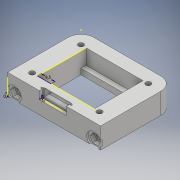
# Autodesk Inventor part: golova 2 prostavka
Saved by Autodesk Inventor 2018.2 (Build 222227000, 227)
## iProperties
Created: 2026-01-20
Part Number: golova 2 prostavka
Material: Типовые
Document SubType Name: Modeling
Designer: Denis
Density: 1 g/cm^3
Appearance: По умолчанию
Author: Denis
## iProperties of the stored document golova 2 prostavka_3DПЕЧАТЬ.ipt
Created: 2026-01-20
Part Number: golova 2 prostavka_3DПЕЧАТЬ
Material: Типовые
Document SubType Name: Modeling
Designer: Denis
Density: 1 g/cm^3
Appearance: По умолчанию
Author: Denis
Autodesk Inventor part; units mm, degrees
ref_plane "YZ Plane" through (0, 0, 0) normal (1, 0, 0) x (0, 1, 0)
ref_plane "XZ Plane" through (0, 0, 0) normal (0, 1, 0) x (-1, 0, 0)
ref_plane "XY Plane" through (0, 0, 0) normal (0, 0, 1) x (1, 0, 0)
sketch "Эскиз1" plane through (0, 0, 0) normal (0, 0, 1) x (1, 0, 0)
  point P0 (0, 0)
sketch "Эскиз2" plane through (0, 0, 0) normal (0, 0, 1) x (1, 0, 0)
  line L0 (0, 0) -> (64.3, 0)
  line L1 (64.3, 0) -> (64.3, -50.7)
  line L2 (64.3, -50.7) -> (0, -50.7)
  line L3 (0, -50.7) -> (0, 0)
  dimension "d0" = 64.3
  dimension "d1" = 50.7
  constraints: 8 end point, 2 parallel, 1 horizontal, 1 perpendicular
  measures "d0" distance of L1.end L2.end
  measures "d1" distance of L0.end L1.end
extrude "Выдавливание1" add sketch "Эскиз2" along normal blind 11.5
sketch "Эскиз3" plane through (0, 0, 11.5) normal (0, 0, 1) x (1, 0, 0)
  line L0 (64.3, 0) -> (0, 0) projected
  line L1 (0, 0) -> (0, -12.4)
  line L2 (0, 0) -> (0, -50.7) projected
  line L3 (0, -12.4) -> (12.4, -12.4)
  line L4 (12.4, -12.4) -> (51.9, -12.4)
  line L5 (51.9, -12.4) -> (51.9, -39.1)
  line L6 (51.9, -39.1) -> (12.4, -39.1)
  line L7 (12.4, -39.1) -> (12.4, -12.4)
  dimension "d4" = 12.4
  dimension "d5" = 12.4
  dimension "d6" = 39.5
  dimension "d7" = 26.7
  constraints: 12 end point, 2 parallel, 2 perpendicular, 1 horizontal, 1 point on line
  measures "d4" distance of L0.end L1.end
  measures "d5" distance of L1.end L3.end
  measures "d6" distance of L5.end L6.end
  measures "d7" distance of L4.end L5.end
extrude "Выдавливание2" cut sketch "Эскиз3" against normal blind 11.5
sketch "Эскиз4" plane through (0, 0, 11.5) normal (0, 0, 1) x (1, 0, 0)
  line L0 (12.4, -39.1) -> (51.9, -39.1) projected
  line L1 (12.4, -39.1) -> (8.8645, -42.6355)
  line L2 (12.4, -39.1) -> (17.4, -39.1) construction
  circle A0 centre (8.8645, -42.6355) radius 1.7
  line L3 (51.9, -12.4) -> (12.4, -12.4) projected
  line L4 (12.4, -12.4) -> (8.8645, -8.8645)
  line L5 (12.4, -12.4) -> (17.4, -12.4) construction
  circle A1 centre (8.8645, -8.8645) radius 1.7
  line L6 (51.9, -39.1) -> (51.9, -12.4) projected
  line L7 (51.9, -12.4) -> (55.4355, -8.8645)
  line L8 (51.9, -12.4) -> (56.9, -12.4) construction
  circle A2 centre (55.4355, -8.8645) radius 1.7
  line L9 (51.9, -39.1) -> (55.4355, -42.6355)
  circle A3 centre (55.4355, -42.6355) radius 1.7
  point P0 (0, 0)
  dimension "d10" = 5
  dimension "d11" = 135
  dimension "d12" = 3.4
  dimension "d13" = 5
  dimension "d14" = 135
  dimension "d15" = 3.4
  dimension "d16" = 5
  dimension "d17" = 45
  dimension "d18" = 3.4
  dimension "d19" = 3.4
  constraints: 14 end point, 4 centre point, 4 coincident, 3 equal length, 3 horizontal
  measures "d10" distance of L0.start L1.end
  measures "d11" angle of L1 L2
  measures "d12" diameter of A0
  measures "d13" distance of L3.end L4.end
  measures "d14" angle of L5 L4
  measures "d15" diameter of A1
  measures "d16" distance of L3.start L7.end
  measures "d17" angle of L8 L7
  measures "d18" diameter of A2
  measures "d19" diameter of A3
extrude "Выдавливание3" cut sketch "Эскиз4" against normal blind 11.5
sketch "Эскиз5" plane through (0, 0, 11.5) normal (0, 0, 1) x (1, 0, 0)
  circle A0 centre (8.8645, -8.8645) radius 1.7 projected
  circle A1 centre (8.8645, -8.8645) radius 1.8
  circle A2 centre (55.4355, -8.8645) radius 1.7 projected
  circle A3 centre (55.4355, -8.8645) radius 1.8
  circle A4 centre (55.4355, -42.6355) radius 1.7 projected
  circle A5 centre (55.4355, -42.6355) radius 1.8
  circle A6 centre (8.8645, -42.6355) radius 1.7 projected
  circle A7 centre (8.8645, -42.6355) radius 1.8
  point P0 (0, 0)
  dimension "d22" = 3.6
  dimension "d23" = 3.6
  dimension "d24" = 3.6
  dimension "d25" = 3.6
  constraints: 4 centre point, 4 coincident
  measures "d22" diameter of A1
  measures "d23" diameter of A3
  measures "d24" diameter of A5
  measures "d25" diameter of A7
extrude "Выдавливание4" cut sketch "Эскиз5" against normal blind 11.5 contours A0 | A3 | A5 | A7
sketch "Эскиз6" plane through (0, 0, 11.5) normal (0, 0, 1) x (1, 0, 0)
  circle A0 centre (8.8645, -8.8645) radius 1.7 projected
  circle A1 centre (8.8645, -8.8645) radius 1.8
  point P0 (0, 0)
  dimension "d28" = 3.6
  constraints: 1 centre point, 1 coincident
  measures "d28" diameter of A1
extrude "Выдавливание5" cut sketch "Эскиз6" against normal blind 11.5 contours A0 | A1
sketch "Эскиз7" plane through (0, 0, 11.5) normal (0, 0, 1) x (1, 0, 0)
  point P0 (0, 0)
sketch "Эскиз8" plane through (0, 0, 11.5) normal (0, 0, 1) x (1, 0, 0)
  line L0 (12.4, -39.1) -> (12.4, -12.4) projected
  line L1 (12.4, -12.4) -> (51.9, -12.4)
  line L2 (51.9, -12.4) -> (51.9, -8.9)
  line L3 (51.9, -8.9) -> (12.4, -8.9)
  line L4 (12.4, -8.9) -> (12.4, -12.4)
  line L5 (51.9, -39.1) -> (12.4, -39.1) projected
  line L6 (12.4, -39.1) -> (51.9, -39.1)
  line L7 (51.9, -39.1) -> (51.9, -42.6)
  line L8 (51.9, -42.6) -> (12.4, -42.6)
  line L9 (12.4, -42.6) -> (12.4, -39.1)
  point P0 (0, 0)
  dimension "d31" = 39.5
  dimension "d32" = 3.5
  dimension "d33" = 39.5
  dimension "d34" = 3.5
  constraints: 16 end point, 4 parallel, 2 horizontal, 2 perpendicular
  measures "d31" distance of L3.end L2.end
  measures "d32" distance of L2.end L1.end
  measures "d33" distance of L7.end L8.end
  measures "d34" distance of L6.end L7.end
extrude "Выдавливание6" cut sketch "Эскиз8" against normal blind 7.5
sketch "Эскиз9" plane through (0, 0, 11.5) normal (0, 0, 1) x (1, 0, 0)
  point P0 (0, 0)
sketch "Эскиз10" plane through (0, 0, 11.5) normal (0, 0, 1) x (1, 0, 0)
  point P0 (0, 0)
fillet "Сопряжение1" radius 9 2 edges at (64.3, 0, 5.75) (0, 0, 5.75)
sketch "Эскиз11" plane through (0, 0, 11.5) normal (0, 0, 1) x (1, 0, 0)
  point P0 (0, 0)
sketch "Эскиз12" plane through (0, -50.7, 0) normal (0, -1, 0) x (1, 0, 0)
  point P0 (0, 0)
sketch "Эскиз13" plane through (0, -50.7, 0) normal (0, -1, 0) x (1, 0, 0)
  line L0 (0, 0) -> (0, 11.5) projected
  line L1 (0, 0) -> (0, 0.6)
  dimension "d38" = 0.6
  constraints: 2 end point, 1 point on line
  measures "d38" distance of L0.start L1.end
sketch "Эскиз14" plane through (0, -50.7, 0) normal (0, -1, 0) x (1, 0, 0)
  line L0 (64.3, 0) -> (0, 0) projected
  line L1 (0, 0) -> (0, 0.8)
  line L2 (0, 0) -> (0, 11.5) projected
  line L3 (0, 0.8) -> (2.8, 0.8)
  line L4 (2.8, 0.8) -> (6.4, 0.8)
  line L5 (6.4, 0.8) -> (8.2, 3.9177)
  line L6 (8.2, 3.9177) -> (6.4, 7.0354)
  line L7 (6.4, 7.0354) -> (2.8, 7.0354)
  line L8 (2.8, 7.0354) -> (1, 3.9177)
  line L9 (1, 3.9177) -> (2.8, 0.8)
  dimension "d39" = 0.8
  dimension "d40" = 2.8
  dimension "d41" = 3.6
  dimension "d42" = 3.6
  dimension "d43" = 120
  dimension "d44" = 3.6
  dimension "d45" = 120
  constraints: 16 end point, 2 parallel, 2 point on line, 1 perpendicular
  measures "d39" distance of L0.end L1.end
  measures "d40" distance of L1.end L3.end
  measures "d41" distance of L3.end L4.end
  measures "d42" distance of L4.end L5.end
  measures "d43" angle of L5 L4
  measures "d44" distance of L5.end L6.end
  measures "d45" angle of L6 L5
extrude "Выдавливание7" cut sketch "Эскиз14" against normal blind 3.8
sketch "Эскиз15" plane through (0, -46.9, 0) normal (0, -1, 0) x (1, 0, 0)
  point P0 (0, 0)
sketch "Эскиз16" plane through (0, -46.9, 0) normal (0, -1, 0) x (1, 0, 0)
  line L0 (1, 3.9177) -> (2.8, 7.0354) projected
  line L1 (1, 3.9177) -> (4.6, 3.9177)
  circle A0 centre (4.6, 3.9177) radius 1.8
  point P0 (0, 0)
  dimension "d48" = 3.6
  constraints: 2 end point, 1 centre point, 1 coincident, 1 horizontal
  measures "d48" diameter of A0
extrude "Выдавливание8" cut sketch "Эскиз16" against normal blind 3
sketch "Эскиз17" plane through (0, -50.7, 0) normal (0, -1, 0) x (1, 0, 0)
  point P0 (0, 0)
sketch "Эскиз18" plane through (0, -50.7, 0) normal (0, -1, 0) x (1, 0, 0)
  line L0 (64.3, 0) -> (0, 0) projected
  line L1 (64.3, 0) -> (61.5, 0)
  line L2 (61.5, 0) -> (61.5, 0.8)
  line L3 (61.5, 0.8) -> (57.9, 0.8)
  line L4 (57.9, 0.8) -> (56.1, 3.9177)
  line L5 (56.1, 3.9177) -> (57.9, 7.0354)
  line L6 (57.9, 7.0354) -> (61.5, 7.0354)
  line L7 (61.5, 7.0354) -> (63.3, 3.9177)
  line L8 (63.3, 3.9177) -> (61.5, 0.8)
  dimension "d51" = 2.8
  dimension "d52" = 0.8
  dimension "d53" = 3.6
  dimension "d54" = 3.6
  dimension "d55" = 120
  dimension "d56" = 3.6
  dimension "d57" = 120
  constraints: 16 end point, 3 parallel, 2 perpendicular, 1 point on line
  measures "d51" distance of L0.start L1.end
  measures "d52" distance of L1.end L2.end
  measures "d53" distance of L2.end L3.end
  measures "d54" distance of L3.end L4.end
  measures "d55" angle of L3 L4
  measures "d56" distance of L4.end L5.end
  measures "d57" angle of L4 L5
extrude "Выдавливание9" cut sketch "Эскиз18" against normal blind 3.8
sketch "Эскиз19" plane through (0, -46.9, 0) normal (0, -1, 0) x (1, 0, 0)
  circle A0 centre (59.7, 3.9177) radius 1.8
  point P0 (0, 0)
  dimension "d60" = 3.6
  constraints: 1 centre point
  measures "d60" diameter of A0
extrude "Выдавливание10" cut sketch "Эскиз19" against normal blind 3
sketch "Эскиз20" plane through (0, -50.7, 0) normal (0, -1, 0) x (1, 0, 0)
  point P0 (0, 0)
sketch "Эскиз21" plane through (0, -50.7, 0) normal (0, -1, 0) x (1, 0, 0)
  point P0 (0, 0)
sketch "Эскиз22" plane through (0, 0, 11.5) normal (0, 0, 1) x (1, 0, 0)
  point P0 (0, 0)
sketch "Эскиз23" plane through (0, 0, 11.5) normal (0, 0, 1) x (1, 0, 0)
  line L0 (24.9297, -42.6112) -> (32.7764, -42.6112)
  line L1 (32.7764, -42.6112) -> (32.7764, -40.2928)
  line L2 (32.7764, -40.2928) -> (24.9297, -40.2928)
  line L3 (24.9297, -40.2928) -> (24.9297, -42.6112)
  point P0 (0, 0)
  constraints: 8 end point, 2 parallel, 1 horizontal, 1 perpendicular
sketch "Эскиз24" plane through (0, 0, 11.5) normal (0, 0, 1) x (1, 0, 0)
  line L0 (0, -50.7) -> (64.3, -50.7) projected
  line L1 (0, -50.7) -> (64.3, -50.7)
  line L2 (64.3, -50.7) -> (64.3, 0)
  line L3 (64.3, 0) -> (0, 0)
  line L4 (0, 0) -> (0, -50.7)
  line L5 (12.4, -42.6) -> (12.4, -8.9) projected
  line L6 (51.9, -8.9) -> (51.9, -42.6) projected
  line L7 (12.4, -42.6) -> (51.9, -42.6)
  line L8 (51.9, -42.6) -> (51.9, -8.9)
  line L9 (51.9, -8.9) -> (12.4, -8.9)
  line L10 (12.4, -8.9) -> (12.4, -42.6)
  constraints: 16 end point, 4 parallel, 2 horizontal, 2 perpendicular
extrude "Выдавливание11" add sketch "Эскиз24" along normal blind 3
fillet "Сопряжение2" radius 9 2 edges at (64.3, 0, 13) (0, 0, 13)
sketch "Эскиз25" plane through (0, 0, 14.5) normal (0, 0, 1) x (1, 0, 0)
  circle A0 centre (8.8645, -8.8645) radius 1.8 projected
  circle A1 centre (8.8645, -8.8645) radius 1.8
  circle A2 centre (55.4355, -8.8645) radius 1.8 projected
  circle A3 centre (55.4355, -8.8645) radius 1.8
  circle A4 centre (55.4355, -42.6355) radius 1.8 projected
  circle A5 centre (55.4355, -42.6355) radius 1.8
  circle A6 centre (8.8645, -42.6355) radius 1.8 projected
  circle A7 centre (8.8645, -42.6355) radius 1.8
  point P0 (0, 0)
  constraints: 4 centre point, 4 coincident
extrude "Выдавливание12" cut sketch "Эскиз25" against normal blind 3
sketch "Эскиз26" plane through (0, 0, 14.5) normal (0, 0, 1) x (1, 0, 0)
  line L0 (12.4, -42.6) -> (12.4, -8.9) projected
  line L1 (12.4, -42.6) -> (21.9, -42.6)
  line L2 (51.9, -42.6) -> (12.4, -42.6) projected
  point P0 (0, 0)
  dimension "d68" = 9.5
  constraints: 2 end point, 1 point on line
  measures "d68" distance of L0.start L1.end
sketch "Эскиз27" plane through (0, -50.7, 0) normal (0, -1, 0) x (1, 0, 0)
  line L0 (12.4, 14.5) -> (51.9, 14.5) projected
  line L1 (12.4, 14.5) -> (21.9, 14.5)
  line L2 (21.9, 14.5) -> (40.7, 14.5)
  line L3 (40.7, 14.5) -> (40.7, 9.5)
  line L4 (40.7, 9.5) -> (21.9, 9.5)
  line L5 (21.9, 9.5) -> (21.9, 14.5)
  point P0 (0, 0)
  dimension "d69" = 9.5
  dimension "d70" = 18.8
  dimension "d71" = 5
  constraints: 10 end point, 2 parallel, 1 horizontal, 1 perpendicular, 1 point on line
  measures "d69" distance of L0.start L1.end
  measures "d70" distance of L3.end L4.end
  measures "d71" distance of L2.end L3.end
extrude "Выдавливание13" cut sketch "Эскиз27" against normal blind 3.5
sketch "Эскиз28" plane through (21.9, -50.7, 9.5) normal (0, 0, 1) x (1, 0, 0)
  line L0 (0, 0) -> (0, 3.5) projected
  line L1 (18.8, 0) -> (18.8, 3.5) projected
  line L2 (0, 3.5) -> (18.8, 3.5)
  line L3 (18.8, 3.5) -> (18.8, 2.5096)
  line L4 (18.8, 2.5096) -> (0, 2.5096)
  line L5 (0, 2.5096) -> (0, 3.5)
  point P0 (-21.9, 50.7)
  constraints: 8 end point, 2 parallel, 1 horizontal, 1 perpendicular, 1 point on line
extrude "Выдавливание14" cut sketch "Эскиз28" against normal blind 1.2
sketch "Эскиз29" plane through (0, -47.2, 0) normal (0, -1, 0) x (1, 0, 0)
  line L0 (40.7, 9.5) -> (21.9, 9.5) projected
  line L1 (21.9, 9.5) -> (23.4, 9.5)
  line L2 (23.4, 9.5) -> (24.4, 9.5)
  line L3 (23.4, 9.5) -> (23.4, 10.5)
  line L4 (23.4, 10.5) -> (39.2, 10.5)
  line L5 (39.2, 10.5) -> (39.2, 12.8)
  line L6 (39.2, 12.8) -> (23.4, 12.8)
  line L7 (23.4, 12.8) -> (23.4, 10.5)
  point P0 (0, 0)
  dimension "d76" = 1.5
  dimension "d77" = 1
  dimension "d78" = 1
  dimension "d79" = 15.8
  dimension "d80" = 2.3
  constraints: 14 end point, 2 parallel, 2 perpendicular, 2 point on line, 1 horizontal
  measures "d76" distance of L0.end L1.end
  measures "d77" distance of L1.end L2.end
  measures "d78" distance of L1.end L3.end
  measures "d79" distance of L6.end L5.end
  measures "d80" distance of L5.end L4.end
extrude "Выдавливание15" cut sketch "Эскиз29" against normal blind 12
fillet "Сопряжение3" radius 2 4 edges at (31.3, -47.2, 12.8) (31.3, -47.2, 10.5) (23.4, -47.2, 11.65) (39.2, -47.2, 11.65)
sketch "Эскиз30" plane through (0, -50.7, 0) normal (0, -1, 0) x (1, 0, 0)
  point P0 (0, 0)
sketch "Эскиз31" plane through (0, 0, 14.5) normal (0, 0, 1) x (1, 0, 0)
  line L0 (40.7, -48.1904) -> (21.9, -48.1904) projected
  line L1 (64.3, -50.7) -> (0, -50.7) projected
  line L2 (21.9, -48.1904) -> (40.7, -48.1904)
  line L3 (40.7, -48.1904) -> (40.7, -50.7)
  line L4 (40.7, -50.7) -> (21.9, -50.7)
  line L5 (21.9, -50.7) -> (21.9, -48.1904)
  point P0 (0, 0)
  dimension "d84" = 18.8
  constraints: 8 end point, 2 parallel, 1 horizontal, 1 perpendicular, 1 point on line
  measures "d84" distance of L3.end L4.end
extrude "Выдавливание16" cut sketch "Эскиз31" against normal blind 5.4
sketch "Эскиз32" plane through (21.9, -50.7, 8.3) normal (0, 0, 1) x (1, 0, 0)
  line L0 (0, 3.5) -> (18.8, 3.5) projected
  line L1 (18.8, 2.5096) -> (0, 2.5096) projected
  line L2 (0, 3.5) -> (18.8, 3.5)
  line L3 (18.8, 3.5) -> (18.8, 2.5096)
  line L4 (18.8, 2.5096) -> (0, 2.5096)
  line L5 (0, 2.5096) -> (0, 3.5)
  point P0 (-21.9, 50.7)
  constraints: 8 end point, 2 parallel, 1 horizontal, 1 perpendicular
extrude "Выдавливание17" cut sketch "Эскиз32" against normal blind 0.3
sketch "Эскиз33" plane through (0, -50.7, 0) normal (0, -1, 0) x (1, 0, 0)
  point P0 (0, 0)
sketch "Эскиз34" plane through (0, -50.7, 0) normal (0, -1, 0) x (1, 0, 0)
  point P0 (0, 0)
sketch "Эскиз35" plane through (0, -50.7, 0) normal (0, -1, 0) x (1, 0, 0)
  circle A0 centre (4.6, 3.9177) radius 1.8 projected
  circle A1 centre (4.6, 3.9177) radius 5
  point P0 (0, 0)
  dimension "d89" = 10
  constraints: 1 centre point, 1 coincident
  measures "d89" diameter of A1
extrude "Выдавливание18" cut sketch "Эскиз35" against normal blind 1
sketch "Эскиз36" plane through (64.3, -50.7, 0) normal (0, -1, 0) x (1, 0, 0)
  circle A0 centre (-4.6, 3.9177) radius 1.8 projected
  circle A1 centre (-4.6, 3.9177) radius 5
  point P0 (-64.3, 0)
  dimension "d92" = 10
  constraints: 1 centre point, 1 coincident
  measures "d92" diameter of A1
extrude "Выдавливание19" cut sketch "Эскиз36" against normal blind 1
sketch "Эскиз37" plane through (40.7, -50.7, 14.5) normal (0, -1, 0) x (1, 0, 0)
  point P0 (-40.7, -14.5)
sketch "Эскиз38" plane through (0, 0, 14.5) normal (0, 0, 1) x (1, 0, 0)
  point P0 (0, 0)
sketch "Эскиз39" plane through (40.7, -50.7, 14.5) normal (0, -1, 0) x (1, 0, 0)
  point P0 (-40.7, -14.5)
sketch "Эскиз40" plane through (40.7, -50.7, 14.5) normal (0, -1, 0) x (1, 0, 0)
  line L0 (-17.3, -4.001) -> (-17.3, -1.6996) projected
  line L1 (-1.5, -4) -> (-17.3, -4) projected
  line L2 (-17.3, -1.6996) -> (-16.3, -1.6996)
  line L3 (-16.3, -1.6996) -> (-16.3, -4)
  line L4 (-16.3, -4) -> (-17.3, -4)
  line L5 (-17.3, -4) -> (-17.3, -1.6996)
  point P0 (-40.7, -14.5)
  dimension "d95" = 1
  constraints: 8 end point, 2 parallel, 1 horizontal, 1 perpendicular, 1 point on line
  measures "d95" distance of L3.end L4.end
sketch "Эскиз41" plane through (0, 0, 14.5) normal (0, 0, 1) x (1, 0, 0)
  line L0 (40.7, -48.1904) -> (21.9, -48.1904) projected
  line L1 (21.9, -48.1904) -> (20.7, -48.1904)
  line L2 (20.7, -48.1904) -> (20.7, -47.2)
  line L3 (20.7, -47.2) -> (21.9, -47.2)
  line L4 (21.9, -47.2) -> (21.9, -48.1904)
  line L5 (40.7, -47.2) -> (40.7, -50.7) projected
  line L6 (40.7, -48.1904) -> (41.9, -48.1904)
  line L7 (41.9, -48.1904) -> (41.9, -47.2)
  line L8 (41.9, -47.2) -> (40.7, -47.2)
  line L9 (40.7, -47.2) -> (40.7, -48.1904)
  point P0 (0, 0)
  dimension "d96" = 1.2
  dimension "d97" = 1.2
  constraints: 16 end point, 4 parallel, 3 point on line, 2 horizontal, 2 perpendicular
  measures "d96" distance of L2.end L3.end
  measures "d97" distance of L8.end L7.end
extrude "Выдавливание20" cut sketch "Эскиз41" against normal blind 6.5
sketch "Эскиз42" plane through (0, 0, 14.5) normal (0, 0, 1) x (1, 0, 0)
  line L0 (41.9, -48.1904) -> (20.7, -48.1904) projected
  line L1 (20.7, -48.1904) -> (21.9, -48.1904)
  line L2 (21.9, -48.1904) -> (21.9, -48.7004)
  line L3 (21.9, -48.7004) -> (20.7, -48.7004)
  line L4 (20.7, -48.7004) -> (20.7, -48.1904)
  line L5 (40.7, -48.1904) -> (40.7, -50.7) projected
  line L6 (40.7, -48.1904) -> (41.9, -48.1904)
  line L7 (41.9, -48.1904) -> (41.9, -48.7004)
  line L8 (41.9, -48.7004) -> (40.7, -48.7004)
  line L9 (40.7, -48.7004) -> (40.7, -48.1904)
  point P0 (0, 0)
  dimension "d100" = 1.2
  dimension "d101" = 0.51
  dimension "d102" = 1.2
  constraints: 16 end point, 4 parallel, 2 horizontal, 2 perpendicular, 1 point on line
  measures "d100" distance of L2.end L3.end
  measures "d101" distance of L1.end L2.end
  measures "d102" distance of L7.end L8.end
extrude "Выдавливание21" cut sketch "Эскиз42" against normal blind 6.5
sketch "Эскиз43" plane through (0, 0, 14.5) normal (0, 0, 1) x (1, 0, 0)
  line L0 (20.7, -47.2) -> (21.9, -47.2)
  line L1 (21.9, -47.2) -> (21.9, -47.71)
  line L2 (21.9, -47.71) -> (20.7, -47.71)
  line L3 (20.7, -47.71) -> (20.7, -47.2)
  line L4 (40.7, -47.2) -> (41.9, -47.2) projected
  line L5 (41.9, -47.2) -> (40.7, -47.2)
  line L6 (40.7, -47.2) -> (40.7, -47.71)
  line L7 (40.7, -47.71) -> (41.9, -47.71)
  line L8 (41.9, -47.71) -> (41.9, -47.2)
  point P0 (0, 0)
  dimension "d105" = 1.2
  dimension "d106" = 0.51
  dimension "d107" = 1.2
  dimension "d108" = 0.51
  constraints: 16 end point, 4 parallel, 2 horizontal, 2 perpendicular
  measures "d105" distance of L1.end L2.end
  measures "d106" distance of L0.end L1.end
  measures "d107" distance of L7.end L6.end
  measures "d108" distance of L6.end L5.end
extrude "Выдавливание22" add sketch "Эскиз43" against normal blind 6.5 contours L4 L8 L7 L6
sketch "Эскиз44" plane through (0, 0, 14.5) normal (0, 0, 1) x (1, 0, 0)
  line L0 (20.7, -48.7004) -> (20.7, -47.2) projected
  line L1 (20.7, -47.2) -> (21.9, -47.2)
  line L2 (21.9, -47.2) -> (21.9, -47.71)
  line L3 (21.9, -47.71) -> (20.7, -47.71)
  line L4 (20.7, -47.71) -> (20.7, -47.2)
  point P0 (0, 0)
  dimension "d111" = 1.2
  dimension "d112" = 0.51
  constraints: 8 end point, 2 parallel, 1 horizontal, 1 perpendicular
  measures "d111" distance of L2.end L3.end
  measures "d112" distance of L1.end L2.end
extrude "Выдавливание23" add sketch "Эскиз44" against normal blind 6.5
sketch "Эскиз45" plane through (0, 0, 14.5) normal (0, 0, 1) x (1, 0, 0)
  point P0 (0, 0)
sketch "Эскиз46" plane through (21.9, -50.7, 8) normal (0, 0, 1) x (1, 0, 0)
  line L0 (0, 3.5) -> (0, 2.99) projected
  line L1 (0, 3.5) -> (18.8, 3.5) projected
  line L2 (0, 2.99) -> (18.8, 2.99)
  line L3 (18.8, 2.99) -> (18.8, 3.5)
  line L4 (18.8, 3.5) -> (0, 3.5)
  line L5 (0, 3.5) -> (0, 2.99)
  point P0 (-21.9, 50.7)
  constraints: 8 end point, 2 parallel, 1 horizontal, 1 perpendicular
extrude "Выдавливание24" add sketch "Эскиз46" along normal blind 0.5
sketch "Эскиз47" plane through (0, 0, 9.1) normal (0, 0, 1) x (1, 0, 0)
  line L0 (21.9, -48.1904) -> (21.9, -48.7004) projected
  line L1 (40.7, -48.7004) -> (40.7, -48.1904) projected
  line L2 (21.9, -48.1904) -> (40.7, -48.1904)
  line L3 (40.7, -48.1904) -> (40.7, -48.7004)
  line L4 (40.7, -48.7004) -> (21.9, -48.7004)
  line L5 (21.9, -48.7004) -> (21.9, -48.1904)
  point P0 (0, 0)
  constraints: 8 end point, 2 parallel, 1 horizontal, 1 perpendicular
extrude "Выдавливание25" cut sketch "Эскиз47" against normal blind 1.1
